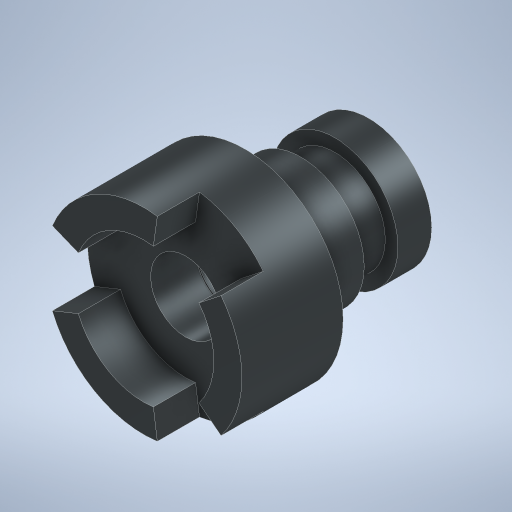
# Autodesk Inventor part: tarea 3 dinamica
Saved by Autodesk Inventor 2023 (Build 270158000, 158)
## iProperties
Created: 2023-05-05
Part Number: tarea 3 dinamica
Material: Iron, Ductile
Document SubType Name: Modeling
Designer: Usuario
Density: 7.15 g/cm^3
Appearance: Iron Gray
Author: Usuario
Autodesk Inventor part; units mm, degrees
ref_plane "YZ Plane" through (0, 0, 0) normal (1, 0, 0) x (0, 1, 0)
ref_plane "XZ Plane" through (0, 0, 0) normal (0, 1, 0) x (-1, 0, 0)
ref_plane "XY Plane" through (0, 0, 0) normal (0, 0, 1) x (1, 0, 0)
sketch "Sketch1" plane through (0, 0, 0) normal (0, 0, 1) x (1, 0, 0)
  circle A0 centre (0, 0) radius 22.5
  constraints: 1 centre point
extrude "Extrusion1" add sketch "Sketch1" along normal blind 12
sketch "Sketch2" plane through (0, 0, 12) normal (0, 0, 1) x (1, 0, 0)
  circle A0 centre (0, 0) radius 18
  constraints: 1 centre point, 1 coincident
extrude "Extrusion2" add sketch "Sketch2" along normal blind 12
sketch "Sketch3" plane through (0, 0, 24) normal (0, 0, 1) x (1, 0, 0)
  circle A0 centre (0, 0) radius 22.5
  constraints: 1 centre point, 1 coincident
extrude "Extrusion3" add sketch "Sketch3" along normal blind 20
sketch "Sketch4" plane through (0, 0, 44) normal (0, 0, 1) x (1, 0, 0)
  circle A0 centre (0, 0) radius 35
  constraints: 1 centre point, 1 coincident
extrude "Extrusion4" add sketch "Sketch4" along normal blind 36
sketch "Sketch5" plane through (0, 0, 80) normal (0, 0, 1) x (1, 0, 0)
  circle A0 centre (0, 0) radius 25
  constraints: 1 centre point, 1 coincident
extrude "Extrusion5" cut sketch "Sketch5" against normal blind 15
sketch "Sketch6" plane through (0, 0, 80) normal (0, 0, 1) x (1, 0, 0)
  circle A0 centre (0, 0) radius 35 projected
  line L0 (0, 0) -> (-32.4578, -13.0955)
  line L1 (0, 0) -> (-32.4578, 13.0955)
  arc A1 (-32.4578, 13.0955) -> (-32.4578, -13.0955) centre (0, 0) ccw
  line L2 (0, 0) -> (27.5699, -21.5615)
  line L3 (0, 0) -> (4.8879, -34.657)
  arc A2 (4.8879, -34.657) -> (27.5699, -21.5615) centre (0, 0) ccw
  line L4 (0, 0) -> (4.8879, 34.657)
  line L5 (0, 0) -> (27.5699, 21.5615)
  arc A3 (27.5699, 21.5615) -> (4.8879, 34.657) centre (0, 0) ccw
  dimension "d17" = 360
  constraints: 12 end point, 8 point on circle, 3 centre point, 3 coincident, 1 concentric, 20 other
extrude "Extrusion6" cut sketch "Sketch6" against normal blind 15 contours L5 L4 A0 | A0 L3 L2 | L0 A0 L1
sketch "Sketch7" plane through (0, 0, 65) normal (0, 0, 1) x (1, 0, 0)
  arc A0 (11.4564, 5) -> (11.4564, -5) centre (0, 0) ccw
  line L0 (18.8783, 0) -> (18.8783, 5)
  line L1 (18.8783, 0) -> (18.8783, -5)
  line L2 (18.8783, -5) -> (11.4564, -5)
  line L3 (18.8783, 5) -> (11.4564, 5)
  constraints: 8 end point, 2 horizontal, 2 point on circle, 2 vertical, 1 centre point, 1 coincident
extrude "Extrusion7" cut sketch "Sketch7" against normal blind 16
sketch "Sketch8" plane through (0, 0, 0) normal (0, 0, -1) x (-1, 0, 0)
  point P0 (0, 0)
sketch "Sketch9" plane through (0, 0, 49) normal (0, 0, 1) x (1, 0, 0)
  circle A0 centre (0, 0) radius 11.9112
  constraints: 1 centre point, 1 coincident
extrude "Extrusion8" cut sketch "Sketch9" against normal blind 50.8
body "Solid1"
